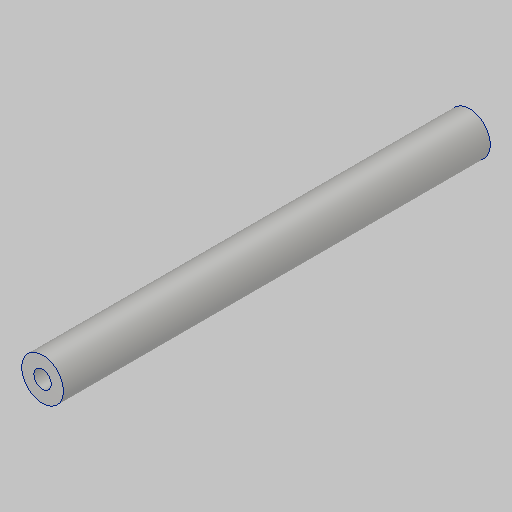
# Autodesk Inventor part: AR-003
Saved by Autodesk Inventor 2023.5 (Build 275446000, 446)
## iProperties
RuleStatus: InUse
Created: 2025-01-22
Part Number: AR-003
Material: Aluminum 6061
Document SubType Name: Modeling
Designer: slick
Density: 2.7 g/cm^3
Appearance: Aluminum - Flat
Mass: 15.4045 g
Surface Area: 42.205 cm^2
Volume: 5.70535 cm^3
AfterDocNew0: Open Form 1
Author: slick
Autodesk Inventor part; units mm, degrees
ref_plane "YZ Plane" through (0, 0, 0) normal (1, 0, 0) x (0, 1, 0)
ref_plane "XZ Plane" through (0, 0, 0) normal (0, 1, 0) x (-1, 0, 0)
ref_plane "XY Plane" through (0, 0, 0) normal (0, 0, 1) x (1, 0, 0)
sketch "Sketch1" plane through (0, 0, 0) normal (0, 0, 1) x (1, 0, 0)
  circle A0 centre (0, 0) radius 4.7625
  dimension "d10" = 9.525
  constraints: 2 coincident, 1 centre point
  measures "d10" diameter of A0
extrude "Extrusion1" add sketch "Sketch1" along normal blind 96.8248
hole "Hole1" at (0, 0, 0) direction (0, 0, 1) diameter 3.9624 end through all thread size "10-32 UNF" class "2B" standard "ANSI Unified Screw Threads"
equation "\"d10\" = OutsideDiameter"
equation "\"d1\" = StandoffLength"
equation "\"StandoffLength\" = 96.8248"
equation "\"HoleDiameter\" = 5.1054"
equation "\"OutsideDiameter\" = 9.525"
body "Solid1"
